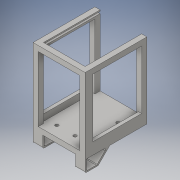
# Autodesk Inventor part: Base
Saved by Autodesk Inventor 2016 (Build 200138000, 138)
## iProperties
Created: 2018-09-29
Part Number: Base
Material: Generic
Document SubType Name: Modeling
Designer: Kyle
Density: 1 g/cm^3
Appearance: Default
Author: Kyle
Autodesk Inventor part; units mm, degrees
ref_plane "YZ Plane" through (0, 0, 0) normal (1, 0, 0) x (0, 1, 0)
ref_plane "XZ Plane" through (0, 0, 0) normal (0, 1, 0) x (-1, 0, 0)
ref_plane "XY Plane" through (0, 0, 0) normal (0, 0, 1) x (1, 0, 0)
sketch "Sketch1" plane through (0, 0, 0) normal (0, 1, 0) x (-1, 0, 0)
  line L0 (-40, -47.5) -> (40, -47.5)
  line L1 (40, -47.5) -> (40, 47.5)
  line L2 (40, 47.5) -> (-40, 47.5)
  line L3 (-40, 47.5) -> (-40, -47.5)
  line L4 (-40, -47.5) -> (40, 47.5) construction
  line L5 (40, -47.5) -> (-40, 47.5) construction
  point P0 (0, 0)
  dimension "d0" = 80
  dimension "d1" = 95
  constraints: 12 end point, 2 midpoint, 2 parallel, 1 horizontal, 1 perpendicular
  measures "d0" distance of L2.end L1.end
  measures "d1" distance of L0.end L1.end
extrude "Extrusion1" add sketch "Sketch1" along normal blind 8
sketch "Sketch2" plane through (40, 0, 47.5) normal (1, 0, 0) x (0, 0, -1)
  line L0 (0, 0) -> (95, 0) projected
  line L1 (95, 0) -> (95, 8) projected
  line L2 (0, 8) -> (95, 8) projected
  line L3 (0, 0) -> (0, 8) projected
  line L4 (95, 0) -> (0, 0) projected
  line L5 (0, 0) -> (0, -16)
  line L6 (2, -18) -> (19.1716, -18)
  line L7 (2, -2) -> (2, -14)
  line L8 (4, -16) -> (17.1716, -16)
  line L9 (20.5858, -17.4142) -> (37.4142, -0.5858)
  line L10 (18.5858, -15.4142) -> (30.5858, -3.4142)
  arc A0 (2, -14) -> (4, -16) centre (4, -14) ccw
  arc A1 (0, -16) -> (2, -18) centre (2, -16) ccw
  arc A2 (19.1716, -18) -> (20.5858, -17.4142) centre (19.1716, -16) ccw
  arc A3 (17.1716, -16) -> (18.5858, -15.4142) centre (17.1716, -14) ccw
  line L11 (4, 0) -> (29.1716, 0)
  arc A4 (30.5858, -3.4142) -> (29.1716, 0) centre (29.1716, -2) ccw
  line L12 (38.8284, 0) -> (47.5, 0)
  arc A5 (38.8284, 0) -> (37.4142, -0.5858) centre (38.8284, -2) ccw
  arc A6 (4, 0) -> (2, -2) centre (4, -2) ccw
  point P0 (0, -18)
  point P1 (20, -18)
  point P2 (22, -16)
  point P3 (38, 0)
  point P4 (34, 0)
  point P5 (34, 0)
  dimension "d4" = 18
  dimension "d5" = 20
  dimension "d6" = 2
  dimension "d7" = 45
  dimension "d8" = 2
  dimension "d9" = 2
  dimension "d10" = 2
  constraints: 16 end point, 15 point on line, 14 point on circle, 14 tangent, 7 centre point, 4 equal radius, 3 perpendicular, 1 collinear, 1 parallel
  measures "d4" distance of L0.start point (0, -18)
  measures "d5" distance of point (0, -18) point (20, -18)
  measures "d6" distance between parallel lines of L5 L7
  measures "d7" angle of L9 L0
  measures "d8" radius of A0
  measures "d9" radius of A4
  measures "d10" radius of A5
extrude "Extrusion2" add sketch "Sketch2" against normal up to surface (80 mm away) contours L0 A6 L7 A0 L8 A3 L10 A4 A5 L9 A2 L6 A1 L5
sketch "Sketch3" plane through (-40, 8, 47.5) normal (0, 0, 1) x (1, 0, 0)
  line L0 (80, 0) -> (0, 0) projected
  line L1 (0, 0) -> (15, 0)
  line L2 (80, 0) -> (65, 0)
  line L3 (80, -26) -> (0, -26) projected
  line L4 (15, 0) -> (65, 0)
  line L5 (65, 0) -> (65, -26)
  line L6 (65, -26) -> (15, -26)
  line L7 (15, -26) -> (15, 0)
  line L8 (15, 0) -> (65, 0)
  line L9 (65, 0) -> (65, -8)
  line L10 (65, -8) -> (15, -8)
  line L11 (15, -8) -> (15, 0)
  line L12 (80, -24) -> (80, 0) projected
  point P0 (40, -8)
  dimension "d13" = 15
  dimension "d15" = 50
  dimension "d16" = 8
  dimension "d41" = 15
  constraints: 20 end point, 4 parallel, 3 point on line, 2 horizontal, 2 perpendicular
  measures "d13" distance of L0.end L1.end
  measures "d15" distance of L9.end L10.end
  measures "d16" distance of L8.end L9.end
  measures "d41" distance between parallel lines of L12 L5
extrude "Extrusion3" cut sketch "Sketch3" against normal blind 39 contours L5 L3 L7 L10
sketch "Sketch4" plane through (0, 8, 0) normal (0, 1, 0) x (1, 0, 0)
  line L0 (40, 47.5) -> (-40, 47.5) projected
  line L1 (-40, 47.5) -> (-40, -47.5) projected
  line L2 (-40, -47.5) -> (40, -47.5) projected
  line L3 (40, -47.5) -> (40, 47.5) projected
  line L4 (40, 47.5) -> (-40, 47.5) projected
  line L5 (-40, -47.5) -> (-35, -47.5)
  line L6 (-35, -47.5) -> (-35, 47.5)
  line L7 (-35, 47.5) -> (-40, 47.5)
  line L8 (-40, 47.5) -> (-40, -47.5)
  line L9 (40, -47.5) -> (35, -47.5)
  line L10 (35, -47.5) -> (35, 47.5)
  line L11 (35, 47.5) -> (40, 47.5)
  line L12 (40, 47.5) -> (40, -47.5)
  line L13 (40, -47.5) -> (32, -47.5)
  line L14 (32, -47.5) -> (32, -39.5)
  line L15 (32, -39.5) -> (40, -39.5)
  line L16 (40, -39.5) -> (40, -47.5)
  line L17 (-40, -47.5) -> (-32, -47.5)
  line L18 (-32, -47.5) -> (-32, -39.5)
  line L19 (-32, -39.5) -> (-40, -39.5)
  line L20 (-40, -39.5) -> (-40, -47.5)
  line L21 (-40, 47.5) -> (-40, -47.5) projected
  line L22 (-40, 47.5) -> (-32, 47.5)
  line L23 (-32, 47.5) -> (-32, 39.5)
  line L24 (-32, 39.5) -> (-40, 39.5)
  line L25 (-40, 39.5) -> (-40, 47.5)
  line L26 (40, 47.5) -> (32, 47.5)
  line L27 (32, 47.5) -> (32, 39.5)
  line L28 (32, 39.5) -> (40, 39.5)
  line L29 (40, 39.5) -> (40, 47.5)
  point P0 (0, 0)
  dimension "d19" = 5
  dimension "d20" = 5
  dimension "d21" = 8
  dimension "d22" = 8
  dimension "d23" = 8
  dimension "d24" = 8
  dimension "d25" = 8
  dimension "d26" = 8
  dimension "d27" = 8
  dimension "d28" = 8
  constraints: 48 end point, 12 parallel, 6 horizontal, 6 perpendicular, 2 point on line
  measures "d19" distance of L7.end L6.end
  measures "d20" distance of L10.end L11.end
  measures "d21" distance of L14.end L15.end
  measures "d22" distance of L13.end L14.end
  measures "d23" distance of L19.end L18.end
  measures "d24" distance of L18.end L17.end
  measures "d25" distance of L23.end L24.end
  measures "d26" distance of L22.end L23.end
  measures "d27" distance of L28.end L27.end
  measures "d28" distance of L27.end L26.end
extrude "Extrusion4" add sketch "Sketch4" along normal blind 10 contours L3 L28 L10 L0 | L3 L15 L10 L28 | L3 L2 L10 L15 | L6 L24 L1 L0 | L6 L19 L1 L24 | L6 L2 L1 L19
sketch "Sketch6" plane through (0, 8, 0) normal (0, 1, 0) x (1, 0, 0)
  line L0 (40, 47.5) -> (-40, 47.5) projected
  line L1 (-40, 47.5) -> (-32, 47.5)
  line L2 (-32, 47.5) -> (-32, 39.5)
  line L3 (-32, 39.5) -> (-40, 39.5)
  line L4 (-40, 39.5) -> (-40, 47.5)
  line L5 (40, 47.5) -> (32, 47.5)
  line L6 (32, 47.5) -> (32, 39.5)
  line L7 (32, 39.5) -> (40, 39.5)
  line L8 (40, 39.5) -> (40, 47.5)
  line L9 (-25, -47.5) -> (-40, -47.5) projected
  line L10 (-40, -47.5) -> (-32, -47.5)
  line L11 (-32, -47.5) -> (-32, -39.5)
  line L12 (-32, -39.5) -> (-40, -39.5)
  line L13 (-40, -39.5) -> (-40, -47.5)
  line L14 (40, -43.5) -> (40, -18.3284) projected
  line L15 (-35, -47.5) -> (35, -47.5) projected
  line L16 (40, -40.5) -> (48.82, -40.5) construction
  line L17 (40, -47.5) -> (32, -47.5)
  line L18 (32, -47.5) -> (32, -35.5)
  line L19 (32, -35.5) -> (40, -35.5)
  line L20 (40, -35.5) -> (40, -47.5)
  line L21 (35, -47.5) -> (35, 47.5) projected
  line L22 (35, -47.5) -> (40, -38.8397)
  line L23 (40, -30.3284) -> (40, -43.5) projected
  line L24 (35, -47.5) -> (45, -47.5) construction
  point P0 (0, 0)
  dimension "d42" = 8
  dimension "d43" = 8
  dimension "d44" = 8
  dimension "d45" = 8
  dimension "d46" = 8
  dimension "d47" = 8
  dimension "d81" = 8
  dimension "d82" = 12
  dimension "d83" = 60
  constraints: 38 end point, 8 parallel, 6 horizontal, 4 perpendicular, 4 point on line, 1 equal length
  measures "d42" distance of L2.end L3.end
  measures "d43" distance of L1.end L2.end
  measures "d44" distance of L7.end L6.end
  measures "d45" distance of L6.end L5.end
  measures "d46" distance of L12.end L11.end
  measures "d47" distance of L11.end L10.end
  measures "d81" distance of L18.end L19.end
  measures "d82" distance of L17.end L18.end
  measures "d83" angle of L24 L22
extrude "Extrusion5" add sketch "Sketch6" along normal blind 100
sketch "Sketch7" plane through (0, 108, 0) normal (0, 1, 0) x (1, 0, 0)
  line L0 (-40, -47.5) -> (-40, -45.5) projected
  line L1 (-32, 47.5) -> (-40, 47.5) projected
  line L2 (-40, -47.5) -> (-32, -47.5)
  line L3 (-32, -47.5) -> (-32, 47.5)
  line L4 (-32, 47.5) -> (-40, 47.5)
  line L5 (-40, 47.5) -> (-40, -47.5)
  line L6 (35, -39.5) -> (40, -39.5) projected
  line L7 (-40, -47.5) -> (40, -47.5)
  line L8 (40, -47.5) -> (40, -39.5)
  line L9 (40, -39.5) -> (-40, -39.5)
  line L10 (-40, -39.5) -> (-40, -47.5)
  line L11 (32, 39.5) -> (32, 47.5) projected
  line L12 (32, 47.5) -> (40, 47.5)
  line L13 (40, 47.5) -> (40, -47.5)
  line L14 (40, -47.5) -> (32, -47.5)
  line L15 (32, -47.5) -> (32, 47.5)
  point P0 (0, 0)
  constraints: 24 end point, 6 parallel, 3 horizontal, 3 perpendicular
extrude "Extrusion6" add sketch "Sketch7" along normal blind 8
sketch "Sketch8" plane through (40, 0, -47.5) normal (0, 0, -1) x (-1, 0, 0)
  line L0 (8, 8) -> (72, 8) projected
  line L1 (8, 8) -> (8, 116) projected
  line L2 (0, 116) -> (8, 116) projected
  line L3 (0, 0) -> (0, 116) projected
  line L4 (0, 0) -> (80, 0) projected
  line L5 (80, 0) -> (80, 116) projected
  line L6 (72, 116) -> (80, 116) projected
  line L7 (72, 8) -> (72, 116) projected
  line L8 (0, 116) -> (8, 116) projected
  line L9 (8, 8) -> (8, 108) projected
  line L10 (0, 116) -> (8, 116)
  line L11 (8, 108) -> (0, 108)
  line L12 (0, 108) -> (0, 116)
  line L13 (0, 108) -> (8, 108) projected
  line L14 (8, 108) -> (8, 111)
  line L15 (8, 8) -> (8, 116) projected
  line L16 (8, 111) -> (4, 111)
  line L17 (4, 111) -> (4, 114)
  line L18 (4, 114) -> (8, 114)
  line L19 (80, 116) -> (0, 116) projected
  line L20 (40, 116) -> (40, 8)
  line L21 (72, 8) -> (8, 8) projected
  line L22 (80, 116) -> (72, 116)
  line L23 (80, 116) -> (72, 116)
  line L24 (80, 116) -> (72, 116)
  line L25 (72, 108) -> (80, 108)
  line L26 (80, 108) -> (80, 116)
  line L27 (80, 108) -> (72, 108)
  line L28 (72, 108) -> (72, 111)
  line L29 (72, 111) -> (76, 111)
  line L30 (76, 111) -> (76, 114)
  line L31 (76, 114) -> (72, 114)
  line L32 (8, 114) -> (72, 114)
  line L33 (72, 111) -> (8, 111)
  line L34 (72, 114) -> (76, 114)
  line L35 (76, 114) -> (76, 111)
  line L36 (76, 111) -> (72, 111)
  line L37 (72, 116) -> (72, 114)
  line L38 (72, 111) -> (72, 108)
  line L39 (8, 116) -> (8, 114)
  line L40 (8, 111) -> (8, 108)
  line L41 (4, 114) -> (8, 114)
  line L42 (4, 111) -> (8, 111)
  line L43 (4, 114) -> (76, 114)
  line L44 (76, 114) -> (76, 111)
  line L45 (76, 111) -> (4, 111)
  line L46 (4, 111) -> (4, 114)
  point P0 (40, 0)
  dimension "d52" = 3
  dimension "d53" = 4
  dimension "d54" = 3
  constraints: 66 end point, 8 symmetric about line, 7 parallel, 7 perpendicular, 4 horizontal, 2 collinear, 2 midpoint, 2 point on line
  measures "d52" distance of L14.end L9.end
  measures "d53" distance of L14.end L16.end
  measures "d54" distance of L16.end L17.end
extrude "Extrusion7" cut sketch "Sketch8" against normal blind 91 contours L33 L1 L32 L20 | L20 L32 L7 L33 | L16 L17 L18 L1 | L7 L31 L30 L29
sketch "Sketch9" plane through (0, 8, 0) normal (0, 1, 0) x (1, 0, 0)
  line L0 (0, -31.5) -> (8.5, -31.5)
  circle A0 centre (8.5, -31.5) radius 2.5
  circle A1 centre (-19.5, -31.5) radius 2.5
  circle A2 centre (-19.5, -31.5) radius 2.5
  line L1 (0, -31.5) -> (-19.5, -31.5)
  line L2 (0, 0) -> (0, -31.5)
  line L3 (0, 0) -> (0, 17.5)
  line L4 (0, 17.5) -> (0, 19)
  line L5 (0, 19) -> (24, 19)
  circle A3 centre (24, 19) radius 2.5
  line L6 (0, 0) -> (2.25, 0)
  line L7 (-27.5, 38.25) -> (28.5, 38.25)
  line L8 (28.5, 38.25) -> (28.5, -36.75)
  line L9 (28.5, -36.75) -> (-27.5, -36.75)
  line L10 (-27.5, -36.75) -> (-27.5, 38.25)
  line L11 (-27.5, 38.25) -> (28.5, -36.75) construction
  line L12 (28.5, 38.25) -> (-27.5, -36.75) construction
  line L13 (-19.5, -31.5) -> (-19.5, -36.75)
  line L14 (25.5, 17) -> (28.5, 17)
  line L15 (28.5, 17) -> (28.5, -36.75)
  point P0 (0.5, 0.75)
  dimension "d63" = 5
  dimension "d61" = 5
  dimension "d62" = 5
  dimension "d64" = 17.5
  dimension "d65" = 8.5
  dimension "d66" = 19.5
  dimension "d67" = 31.5
  dimension "d68" = 24
  dimension "d69" = 43.5
  dimension "d70" = 2.25
  dimension "d71" = 56
  dimension "d72" = 75
  dimension "d73" = 5.25
  dimension "d74" = 3
  constraints: 32 end point, 6 horizontal, 5 vertical, 4 perpendicular, 3 centre point, 2 midpoint, 2 parallel, 2 point on line, 1 coincident, 1 concentric, 4 other
  measures "d61" diameter of A0
  measures "d62" diameter of A1
  measures "d64" distance of L3.start L4.start
  measures "d65" distance of L0.start L0.end
  measures "d66" distance of L0.start L1.end
  measures "d67" distance of L3.start L0.start
  measures "d68" distance of L4.end L5.end
  measures "d69" horizontal distance of A1.centre L5.end
  measures "d70" distance of L6.start L6.end
  measures "d71" distance of L11.end L10.start
  measures "d72" distance of L11.end L12.start
  measures "d73" distance of L1.end L13.end
  measures "d74" distance of L14.start L14.end
extrude "Extrusion8" cut sketch "Sketch9" against normal blind 10 contours A0 | L1 L13 A1 | A1 L13 L1 | A3
body "Solid1"
